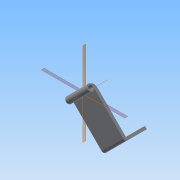
# Autodesk Inventor part: clapet
Saved by Autodesk Inventor 2015 (Build 190159000, 159)
## iProperties
Created: 2015-06-18
Part Number: clapet
Material: Générique
Document SubType Name: Modeling
Designer: Gregwar
Density: 1 g/cm^3
Appearance: Par défaut
Author: Gregwar
Autodesk Inventor part; units mm, degrees
ref_plane "YZ Plane" through (0, 0, 0) normal (1, 0, 0) x (0, 1, 0)
ref_plane "XZ Plane" through (0, 0, 0) normal (0, 1, 0) x (-1, 0, 0)
ref_plane "XY Plane" through (0, 0, 0) normal (0, 0, 1) x (1, 0, 0)
sketch "Esquisse1" plane through (0, 0, 0) normal (0, 1, 0) x (-1, 0, 0)
  line L0 (35, 35) -> (35, 14)
  line L1 (35, 14) -> (42, 10)
  line L2 (42, 10) -> (42, 0)
  line L3 (35, 35) -> (0, 0)
  line L4 (42, 0) -> (0, 0) construction
  line L5 (35, -35) -> (35, -14)
  line L6 (35, -14) -> (42, -10)
  line L7 (42, -10) -> (42, 0)
  line L8 (35, -35) -> (0, 0)
  line L9 (38.5, -12) -> (38.5, 12) construction
  circle A0 centre (38.5, 0) radius 2.15
  circle A1 centre (38.5, 6) radius 2.15
  circle A2 centre (38.5, -6) radius 2.15
  dimension "d0" = 90
  dimension "d1" = 70
  dimension "d4" = 6
  dimension "d11" = 6
  dimension "d16" = 4.3
  dimension "d17" = 20
  dimension "d18" = 4
  dimension "d19" = 7
  constraints: 20 end point, 3 centre point, 3 midpoint, 3 symmetric about line, 3 vertical, 1 horizontal, 1 parallel, 4 other
  measures "d0" angle of L3 L8
  measures "d1" distance of L0.start L5.start
  measures "d4" distance of A0.centre A1.centre
  measures "d11" distance of A0.centre A2.centre
  measures "d16" diameter of A0
  measures "d17" distance of L1.end L6.end
  measures "d18" vertical distance of L1.end L0.end
  measures "d19" distance between parallel lines of L5 L7
extrude "Extrusion1" add sketch "Esquisse1" along normal blind 3
pattern_circular "Réseau circulaire1" count 4 over 360 about axis through (0, 0, 0) along (0, 1, 0) of "Extrusion1"
ref_plane "Plan de construction2" through (0, 0, -14) normal (1, 0, 0) x (0, 0, -1)
ref_plane "Plan de construction3" through (-14, 0, 0) normal (0, 0, -1) x (-1, 0, 0)
chamfer "Chanfrein1" distance 10 angle 45 4 edges at (-35, 1.5, -35) (-35, 1.5, 35) (35, 1.5, -35) (35, 1.5, 35)
sketch "Esquisse3" plane through (0, 0, 0) normal (0, -1, 0) x (1, 0, 0)
  circle A0 centre (0, 38.5) radius 2.15 construction
  circle A1 centre (6, 38.5) radius 2.15 construction
  circle A2 centre (-6, 38.5) radius 2.15 construction
  circle A3 centre (38.5, 6) radius 2.15 construction
  circle A4 centre (38.5, -6) radius 2.15 construction
  circle A5 centre (38.5, 0) radius 2.15 construction
  circle A6 centre (6, -38.5) radius 2.15 construction
  circle A7 centre (-6, -38.5) radius 2.15 construction
  circle A8 centre (0, -38.5) radius 2.15 construction
  circle A9 centre (-38.5, -6) radius 2.15 construction
  circle A10 centre (-38.5, 6) radius 2.15 construction
  circle A11 centre (-38.5, 0) radius 2.15 construction
  line L0 (-35, 25) -> (-35, 14) construction
  line L1 (-35, 14) -> (-42, 10) construction
  line L2 (-42, 10) -> (-42, -10) construction
  line L3 (-42, -10) -> (-35, -14) construction
  line L4 (-35, -14) -> (-35, -25) construction
  line L5 (-25, -35) -> (-14, -35) construction
  line L6 (-14, -35) -> (-10, -42) construction
  line L7 (-10, -42) -> (10, -42) construction
  line L8 (10, -42) -> (14, -35) construction
  line L9 (14, -35) -> (25, -35) construction
  line L10 (35, -25) -> (35, -14) construction
  line L11 (35, -14) -> (42, -10) construction
  line L12 (42, -10) -> (42, 10) construction
  line L13 (42, 10) -> (35, 14) construction
  line L14 (35, 14) -> (35, 25) construction
  line L15 (25, 35) -> (14, 35) construction
  line L16 (14, 35) -> (10, 42) construction
  line L17 (10, 42) -> (-10, 42) construction
  line L18 (-10, 42) -> (-14, 35) construction
  line L19 (-14, 35) -> (-25, 35) construction
  line L20 (-51.72, -12.8291) -> (-12.8291, -51.72)
  line L21 (-12.8291, -51.72) -> (-10, -42)
  line L22 (-42, -10) -> (-51.72, -12.8291)
  line L23 (-35, -14) -> (-42, -10)
  line L24 (-42, -10) -> (-35, -14) projected
  line L25 (-10, -42) -> (-14, -35)
  line L26 (-14, -35) -> (-10, -42) projected
  line L27 (25, 35) -> (35, 25) projected
  line L28 (-35, 25) -> (-25, 35) projected
  line L29 (-25, -35) -> (-35, -25) projected
  line L30 (35, -25) -> (25, -35) projected
  line L31 (-14, -35) -> (-35, -14)
  point P0 (0, 0)
  dimension "d32" = 135
  dimension "d33" = 55
  constraints: 12 end point, 1 collinear, 1 equal length, 1 point on line
  measures "d32" angle of L5 L20
  measures "d33" distance of L20.start L20.end
extrude "Extrusion3" add sketch "Esquisse3" against normal blind 3
sketch "Esquisse4" plane through (-51.72, 0, -12.8291) normal (-0.7071068, 0, -0.7071068) x (-0.7071068, 0, 0.7071068)
  line L0 (0, 0) -> (-55, 0) construction
  line L1 (0, 0) -> (0, 3) construction
  line L2 (-55, 3) -> (0, 3) construction
  line L3 (-55, 0) -> (-55, 3) construction
  line L4 (0, 0) -> (-55, 0)
  line L5 (-55, 0) -> (-55, 24)
  line L6 (-55, 24) -> (0, 24)
  line L7 (0, 24) -> (0, 0)
  point P0 (-27.5, 0)
  dimension "d36" = 24
  constraints: 8 end point, 2 parallel, 1 horizontal, 1 perpendicular
  measures "d36" distance of L4.end L5.end
extrude "Extrusion4" add sketch "Esquisse4" along normal blind 3
sketch "Esquisse5" plane through (-53.8413, 0, -14.9504) normal (-0.7071068, 0, -0.7071068) x (-0.7071068, 0, 0.7071068)
  line L0 (-55, 0) -> (0, 0) construction
  line L1 (0, 0) -> (0, 24) construction
  line L2 (0, 24) -> (-55, 24) construction
  line L3 (-55, 24) -> (-55, 0) construction
  line L4 (0, 0) -> (0, 24) construction
  line L5 (0, 9.2801) -> (-55, 9.2801) construction
  circle A0 centre (-15.1412, 9.2801) radius 7.3571
  line L6 (-27.5, 0) -> (-27.5, 24) construction
  circle A1 centre (-39.8588, 9.2801) radius 7.3571
  constraints: 4 end point, 3 point on line, 2 centre point, 1 midpoint, 1 perpendicular, 1 symmetric about line, 1 other
extrude "Extrusion5" cut sketch "Esquisse5" against normal blind 1
pattern_circular "Réseau circulaire2" count 4 over 360 about axis through (0, 0, 0) along (0, -1, 0) of "Extrusion3", "Extrusion4"
fillet "Congé1" radius 3 2 edges at (-34.3959, 0, 34.3959) (34.3959, 0, -34.3959)
sketch "Esquisse6" plane through (0, 0, 0) normal (0, -1, 0) x (1, 0, 0)
  line L0 (51.72, -12.8291) -> (12.8291, -51.72) construction
  line L1 (51.72, -12.8291) -> (42, -10) construction
  line L2 (42, -10) -> (42, 10) construction
  line L3 (42, 10) -> (51.72, 12.8291) construction
  line L4 (51.72, 12.8291) -> (53.8413, 14.9504) construction
  line L5 (14.9504, 53.8413) -> (53.8413, 14.9504) construction
  line L6 (12.8291, 51.72) -> (14.9504, 53.8413) construction
  line L7 (12.8291, 51.72) -> (10, 42) construction
  line L8 (10, 42) -> (-10, 42) construction
  line L9 (-10, 42) -> (-12.8291, 51.72) construction
  line L10 (-51.72, 12.8291) -> (-12.8291, 51.72) construction
  line L11 (-51.72, 12.8291) -> (-42, 10) construction
  line L12 (-42, 10) -> (-42, -10) construction
  line L13 (-42, -10) -> (-51.72, -12.8291) construction
  line L14 (-51.72, -12.8291) -> (-53.8413, -14.9504) construction
  line L15 (-14.9504, -53.8413) -> (-53.8413, -14.9504) construction
  line L16 (-12.8291, -51.72) -> (-14.9504, -53.8413) construction
  line L17 (-12.8291, -51.72) -> (-10, -42) construction
  line L18 (-10, -42) -> (10, -42) construction
  line L19 (10, -42) -> (12.8291, -51.72) construction
  circle A0 centre (0, 38.5) radius 2.15 construction
  circle A1 centre (6, 38.5) radius 2.15 construction
  circle A2 centre (-6, 38.5) radius 2.15 construction
  circle A3 centre (38.5, 6) radius 2.15 construction
  circle A4 centre (38.5, -6) radius 2.15 construction
  circle A5 centre (38.5, 0) radius 2.15 construction
  circle A6 centre (6, -38.5) radius 2.15 construction
  circle A7 centre (-6, -38.5) radius 2.15 construction
  circle A8 centre (0, -38.5) radius 2.15 construction
  circle A9 centre (-38.5, -6) radius 2.15 construction
  circle A10 centre (-38.5, 6) radius 2.15 construction
  circle A11 centre (-38.5, 0) radius 2.15 construction
  line L20 (14.9504, -53.8413) -> (53.8413, -14.9504) construction
  line L21 (22.0215, -46.7702) -> (-16.8694, -7.8793)
  line L22 (-16.8694, -7.8793) -> (7.8793, 16.8694)
  line L23 (7.8793, 16.8694) -> (46.7702, -22.0215)
  line L24 (46.7702, -22.0215) -> (22.0215, -46.7702)
  line L25 (-16.8694, -7.8793) -> (-13.3339, -11.4149) construction
  line L26 (-13.3339, -11.4149) -> (11.4149, 13.3339) construction
  line L27 (11.4149, 13.3339) -> (7.8793, 16.8694) construction
  line L28 (-4.495, 4.495) -> (34.3959, -34.3959) construction
  line L29 (-13.3339, -11.4149) -> (-30.7818, -28.8628) construction
  circle A12 centre (-15.4552, -13.5362) radius 1.7
  circle A13 centre (-18.9907, -17.0717) radius 1.7
  circle A14 centre (13.5362, 15.4552) radius 1.7
  circle A15 centre (17.0717, 18.9907) radius 1.7
  point P0 (0, 0)
  dimension "d48" = 35
  dimension "d49" = 55
  dimension "d54" = 35
  dimension "d69" = 5
  dimension "d70" = 3
  dimension "d71" = 3.4
  dimension "d74" = 5
  constraints: 18 end point, 4 centre point, 4 perpendicular, 3 collinear, 3 midpoint, 3 point on line, 2 symmetric about line, 1 parallel, 5 other
  measures "d48" distance of L21.end L22.end
  measures "d49" distance of L21.start L21.end
  measures "d54" distance of L25.end L26.end
  measures "d69" distance between parallel lines of L26 L22
  measures "d70" distance from line of A12.centre L21
  measures "d71" diameter of A12
  measures "d74" distance of A12.centre A13.centre
extrude "Extrusion6" cut sketch "Esquisse6" against normal through all contours L21 L22 L23 L24 keep common part
sketch "Esquisse7" plane through (19.9002, 3, -44.6489) normal (-0.7071068, 0, -0.7071068) x (-0.7071068, 0, 0.7071068)
  circle A0 centre (47, -5.5) radius 3.5
  line L0 (47, -3) -> (47, -5.5) construction
  line L1 (0, -3) -> (52, -3) construction
  point P0 (45.6431, -3)
  point P1 (47, -3)
  dimension "d97" = 2.5
  dimension "d98" = 7
  constraints: 2 end point, 1 centre point, 1 perpendicular, 1 vertical
  measures "d97" distance of L0.start L0.end
  measures "d98" diameter of A0
extrude "Extrusion7" add sketch "Esquisse7" against normal blind 35
sketch "Esquisse8" plane through (19.9002, 3, -44.6489) normal (-0.7071068, 0, -0.7071068) x (-0.7071068, 0, 0.7071068)
  arc A0 (43.5, -3) -> (50.5, -3) centre (47, -3) ccw projected
  line L0 (49.4495, -3) -> (52, -3) projected
  line L1 (52, -3) -> (52, 0) projected
  line L2 (52, 0) -> (0, 0) projected
  line L3 (0, 0) -> (0, 21) projected
  line L4 (0, 21) -> (-3, 21) projected
  line L5 (-3, 21) -> (-3, 0) projected
  arc A1 (-3, 0) -> (0, -3) centre (0, 0) ccw projected
  line L6 (0, -3) -> (44.5505, -3) projected
  arc A2 (44.5505, -3) -> (49.4495, -3) centre (47, -5.5) ccw projected
  arc A3 (44.5505, -3) -> (49.4495, -3) centre (47, -5.5) ccw projected
  circle A4 centre (47, -5.5) radius 2.3
  point P0 (45.6431, -3)
  dimension "d99" = 4.6
  constraints: 1 centre point, 1 coincident
  measures "d99" diameter of A4
extrude "Extrusion8" cut sketch "Esquisse8" against normal through all contours A4 A0 | A0 A4
sketch "Esquisse11" plane through (19.9002, 3, -44.6489) normal (-0.7071068, 0, -0.7071068) x (-0.7071068, 0, 0.7071068)
  line L0 (49.4495, -3) -> (52, -3) projected
  line L1 (52, -3) -> (52, 0) projected
  line L2 (52, 0) -> (0, 0) projected
  line L3 (0, 0) -> (0, 21) projected
  line L4 (0, 21) -> (-3, 21) projected
  line L5 (-3, 21) -> (-3, 0) projected
  arc A0 (-3, 0) -> (0, -3) centre (0, 0) ccw projected
  line L6 (0, -3) -> (44.5505, -3) projected
  arc A1 (44.5505, -3) -> (49.4495, -3) centre (47, -5.5) ccw projected
  line L7 (49.4495, -3) -> (49, 0) construction
  line L8 (52, 0) -> (0, 0) projected
  line L9 (49, 0) -> (42, 0) construction
  spline S0 degree 2 poles (49.4495, -3) (49, 0) (42, 0) knots 1 1 1 2 2 2
  point P0 (45.6431, -3)
  dimension "d100" = 3
  dimension "d101" = 10
  constraints: 2 point on line, 3 other
  measures "d100" distance of L1.end L7.end
  measures "d101" distance from line of L1 L9.end
extrude "Extrusion9" cut sketch "Esquisse11" against normal through all contours A1 L6 A0 L5 L4 L3 L2 S0 keep common part
fillet "Congé4" radius 4 1 edges at (-2.6915, 0, 2.6915)
sketch "Esquisse12" plane through (0, 0, 0) normal (0, -1, 0) x (1, 0, 0)
  line L0 (19.9002, -44.6489) -> (-11.6018, -13.1469) projected
  line L1 (44.6489, -19.9002) -> (19.9002, -44.6489) projected
  line L2 (13.1469, 11.6018) -> (44.6489, -19.9002) projected
  line L3 (22.0215, -46.7702) -> (46.7702, -22.0215) construction
  line L4 (34.3959, -34.3959) -> (-3.4344, 3.4344) construction
  line L5 (-15.8087, -8.94) -> (8.94, 15.8087) construction
  line L6 (-15.8087, -8.94) -> (8.94, 15.8087) projected
  line L7 (-15.3138, -8.445) -> (22.5165, -46.2752)
  line L8 (8.445, 15.3138) -> (46.2752, -22.5165)
  line L9 (22.5165, -46.2752) -> (22.0215, -46.7702)
  line L10 (22.0215, -46.7702) -> (-15.8087, -8.94)
  line L11 (-15.8087, -8.94) -> (-15.3138, -8.445)
  line L12 (46.2752, -22.5165) -> (46.7702, -22.0215)
  line L13 (46.7702, -22.0215) -> (8.94, 15.8087)
  line L14 (8.94, 15.8087) -> (8.445, 15.3138)
  line L15 (13.1469, 11.6018) -> (-11.6018, -13.1469) projected
  point P0 (-9.0912, -12.122)
  dimension "d91" = 0.7
  constraints: 18 end point, 3 collinear, 2 midpoint, 2 parallel, 2 perpendicular, 2 point on line, 2 symmetric about line
  measures "d91" distance between parallel lines of L0 L7
extrude "Extrusion10" cut sketch "Esquisse12" along normal through all both and the other way through all contours L0 L15 L7 L1 | L1 L7 L9 L10 | L10 L6 L7 L15 | L8 L15 L2 L1 | L1 L13 L12 L8 | L8 L6 L13 L15
